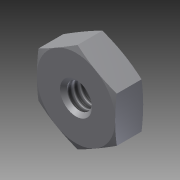
# Autodesk Inventor part: D-3745
Saved by Autodesk Inventor 2012 (Build 160160000, 160)
## iProperties
Created: 2013-01-17
Part Number: D-3745
Material: Default
Catalog Web Link: www.cadenas.de
Description: Mounting Nut for Original Line Cylinders-
Vendor: BIMBA
Document SubType Name: Modeling
Designer: William
Manufacturer: BIMBA
Density: 1 g/cm^3
Category: PARTsolutions
Company: BIMBA
Title: D-3745
Author: Cadenas PARTsolutions
PSOL_IDENT_0: {\\10.0.0.242\data_v9\23d-libs\bimba\bimba\bimba_imperial\bimba_full_line\original_line_cylinders\ac
PSOL_IDENT_1: cessories\mounting_nut.prj},192 {VTYP=3D},{NB=D-3745},{LINA=D-3745},{NN=Mounting Nut for Original Li
PSOL_IDENT_2: ne Cylinders},{DATE=11.06.2012 07:31:25},{GEOMDATE=10.11.2011 00:00:00},{VERSION=},{LINEID=270},{LIN
PSOL_IDENT_3: ESUBID=-1},{WBVAR=MAT}  {NB=D-3745},{LINA=D-3745},{KT=DUMMY},{PN=D-3745},{PN1=D-3745},{C=#5-40},{TH=
PSOL_IDENT_4: UNC},{MAT=},{MAT1='','Zinc-Plated Carbon Steel'},{A=0.31},{A1=0.30700000},{B=0.11},{B1=0.11000000},{
PSOL_IDENT_5: NDM=0.12500000},{PITCH=0.0250},{DIA=-},{DIA2=-},{DIA3=-},{DIA1=0},{DIA4=0.00000000},{DIA5=0.00000000
PSOL_IDENT_6: },{T=-},{T2=-},{T3=-},{T1=0},{T4=0.00000000},{T5=0.00000000},{COLOR=0.75,0.75,0.75,0.00},{TT=0.05000
PSOL_IDENT_7: 000},{TO=0.15000000},{PRA=1}
CNS_NB: D-3745
CNS_NBSYN: $PN.
CNS_LINA: D-3745
CNS_PN: D-3745
CNS_PN1: D-3745
CNS_C: #5-40
CNS_TH: UNC
CNS_MAT: Zinc-Plated Carbon Steel
CNS_MAT1: '','Zinc-Plated Carbon Steel'
CNS_A: 0.31
CNS_A1: 0.30700000
CNS_B: 0.11
CNS_B1: 0.11000000
CNS_NDM: 0.12500000
CNS_PITCH: 0.0250
CNS_DIA: -
CNS_DIA2: -
CNS_DIA3: -
CNS_DIA1: 0.000
CNS_DIA4: 0.00000000
CNS_DIA5: 0.00000000
CNS_T: -
CNS_T2: -
CNS_T3: -
CNS_T1: 0.000
CNS_T4: 0.00000000
CNS_T5: 0.00000000
CNS_COLOR: 0.75,0.75,0.75,0.00
CNS_TT: 0.05000000
CNS_TO: 0.15000000
CNS_PRA: 1
SUPPLIER: BIMBA
ARTICLENO: D-3745
BOMINFO: D-3745
CREATOR: CADENAS GmbH
Autodesk Inventor part; units mm, degrees
sketch "Sketch_8" plane through (0, 0, 0) normal (1, 0, 0) x (0, 1, 0)
  line L0 (0, -2.794) -> (0, 0)
  line L1 (0, 0) -> (3.8989, 0)
  line L2 (3.8989, 0) -> (4.6787, -0.2089)
  line L3 (4.6787, -0.2089) -> (4.6787, -2.5851)
  line L4 (4.6787, -2.5851) -> (3.8989, -2.794)
  line L5 (3.8989, -2.794) -> (0, -2.794)
  line L6 (0, -2.794) -> (0, 0)
  constraints: 14 end point
sketch "Sketch_10" plane through (0, 0, 0) normal (0, 0, 1) x (1, 0, 0)
  line L0 (-7.7978, 7.7978) -> (-7.7978, -7.7978)
  line L1 (-7.7978, -7.7978) -> (7.7978, -7.7978)
  line L2 (7.7978, -7.7978) -> (7.7978, 7.7978)
  line L3 (7.7978, 7.7978) -> (-7.7978, 7.7978)
  line L4 (-3.8989, 2.251) -> (-3.8989, -2.251)
  line L5 (-3.8989, -2.251) -> (0, -4.5021)
  line L6 (0, -4.5021) -> (3.8989, -2.251)
  line L7 (3.8989, -2.251) -> (3.8989, 2.251)
  line L8 (3.8989, 2.251) -> (0, 4.5021)
  line L9 (0, 4.5021) -> (-3.8989, 2.251)
  constraints: 20 end point
revolve "Revolution1" add sketch "Sketch_8" angle 360 about axis through (0, 0, -2.794) along (0, 0, -1)
extrude "Extrusion1" cut sketch "Sketch_10" against normal blind 2.794
sketch "Sketch_13" plane through (0, 0, 0) normal (1, 0, 0) x (0, 1, 0)
  line L0 (0, -2.794) -> (0, 0)
  line L1 (0, 0) -> (1.5875, 0)
  line L2 (1.5875, 0) -> (1.2433, -0.3442)
  line L3 (1.2433, -0.3442) -> (1.2433, -2.4498)
  line L4 (1.2433, -2.4498) -> (1.5875, -2.794)
  line L5 (1.5875, -2.794) -> (0, -2.794)
  line L6 (0, -2.794) -> (0, 0)
  constraints: 14 end point
revolve "Revolution2" cut sketch "Sketch_13" angle 360 about axis through (0, 0, -2.794) along (0, 0, -1)
thread "Thread1" size "5-40 UNC" class "2B" standard "ANSI Unified Screw Threads" full length
ref_plane "NUT_XY" through (0, 0, 0) normal (0, 0, 1) x (1, 0, 0)
ref_plane "NUT_YZ" through (0, 0, 0) normal (1, 0, 0) x (0, 1, 0)
ref_plane "NUT_ZX" through (0, 0, 0) normal (0, 1, 0) x (0, 0, 1)
ref_plane "a1_XY" through (-3.8989, 3.8989, 0) normal (0, 0, 1) x (1, 0, 0)
ref_plane "a1_YZ" through (-3.8989, 3.8989, 0) normal (1, 0, 0) x (0, 1, 0)
ref_plane "a1_ZX" through (-3.8989, 3.8989, 0) normal (0, 1, 0) x (0, 0, 1)
ref_plane "a2_XY" through (3.8989, 3.8989, 0) normal (0, 0, 1) x (1, 0, 0)
ref_plane "a2_YZ" through (3.8989, 3.8989, 0) normal (1, 0, 0) x (0, 1, 0)
ref_plane "a2_ZX" through (3.8989, 3.8989, 0) normal (0, 1, 0) x (0, 0, 1)
ref_plane "b1_XY" through (0, 3.8989, 0) normal (1, 0, 0) x (0, 0, -1)
ref_plane "b1_YZ" through (0, 3.8989, 0) normal (0, 0, -1) x (0, 1, 0)
ref_plane "b1_ZX" through (0, 3.8989, 0) normal (0, 1, 0) x (1, 0, 0)
ref_plane "b2_XY" through (0, 3.8989, -2.794) normal (1, 0, 0) x (0, 0, -1)
ref_plane "b2_YZ" through (0, 3.8989, -2.794) normal (0, 0, -1) x (0, 1, 0)
ref_plane "b2_ZX" through (0, 3.8989, -2.794) normal (0, 1, 0) x (1, 0, 0)
ref_plane "e_XY" through (0, 0, -2.794) normal (1, 0, 0) x (0, 0, -1)
ref_plane "e_YZ" through (0, 0, -2.794) normal (0, 0, -1) x (0, 1, 0)
ref_plane "e_ZX" through (0, 0, -2.794) normal (0, 1, 0) x (1, 0, 0)
ref_plane "th1_XY" through (0, 1.5875, -2.794) normal (1, 0, 0) x (0, 0, -1)
ref_plane "th1_YZ" through (0, 1.5875, -2.794) normal (0, 0, -1) x (0, 1, 0)
ref_plane "th1_ZX" through (0, 1.5875, -2.794) normal (0, 1, 0) x (1, 0, 0)
ref_plane "th2_XY" through (0, -1.5875, -2.794) normal (1, 0, 0) x (0, 0, -1)
ref_plane "th2_YZ" through (0, -1.5875, -2.794) normal (0, 0, -1) x (0, 1, 0)
ref_plane "th2_ZX" through (0, -1.5875, -2.794) normal (0, 1, 0) x (1, 0, 0)
ref_plane "ol1_XY" through (0, 0, -3.8989) normal (0, 1, 0) x (1, 0, 0)
ref_plane "ol1_YZ" through (0, 0, -3.8989) normal (1, 0, 0) x (0, 0, -1)
ref_plane "ol1_ZX" through (0, 0, -3.8989) normal (0, 0, -1) x (0, 1, 0)
ref_plane "ol2_XY" through (2.794, 0, -3.8989) normal (0, 1, 0) x (1, 0, 0)
ref_plane "ol2_YZ" through (2.794, 0, -3.8989) normal (1, 0, 0) x (0, 0, -1)
ref_plane "ol2_ZX" through (2.794, 0, -3.8989) normal (0, 0, -1) x (0, 1, 0)
body "Solid1"
